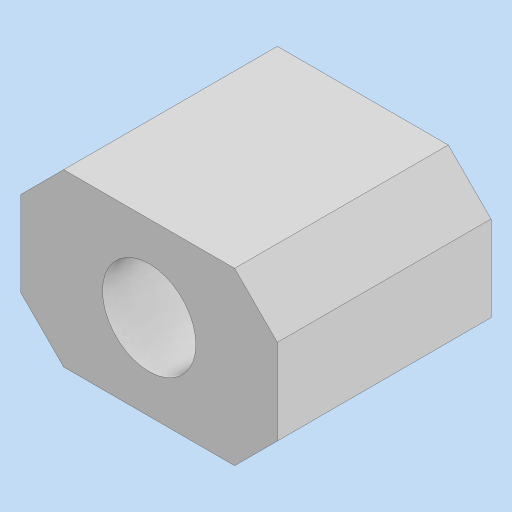
# Autodesk Inventor part: conexion-engrane-hombro
Saved by Autodesk Inventor 2024 (Build 280153000, 153)
## iProperties
Created: 2024-09-11
Part Number: conexion-engrane-hombro
Material: Generic
Document SubType Name: Modeling
Designer: MxMon
Density: 1 g/cm^3
Appearance: Default
Author: MxMon
Autodesk Inventor part; units mm, degrees
ref_plane "YZ Plane" through (0, 0, 0) normal (1, 0, 0) x (0, 1, 0)
ref_plane "XZ Plane" through (0, 0, 0) normal (0, 1, 0) x (-1, 0, 0)
ref_plane "XY Plane" through (0, 0, 0) normal (0, 0, 1) x (1, 0, 0)
sketch "Sketch1" plane through (0, 0, 0) normal (0, 0, 1) x (1, 0, 0)
  line L0 (-6, 4) -> (6, 4)
  line L1 (6, 4) -> (6, -4)
  line L2 (6, -4) -> (-6, -4)
  line L3 (-6, -4) -> (-6, 4)
  line L4 (-6, 4) -> (6, -4) construction
  line L5 (6, 4) -> (-6, -4) construction
  point P0 (0, 0)
  dimension "d0" = 12
  dimension "d1" = 8
  constraints: 12 end point, 2 midpoint, 2 parallel, 1 horizontal, 1 perpendicular
  measures "d0" distance of L1.end L2.end
  measures "d1" distance of L0.end L1.end
extrude "Extrusion1" add sketch "Sketch1" along normal mid plane 10
chamfer "Chamfer1" distance 2 angle 45 4 edges at (6, 4, 0) (-6, 4, 0) (-6, -4, 0) (6, -4, 0)
sketch "Sketch2" plane through (0, 0, -5) normal (0, 0, -1) x (-1, 0, 0)
  circle A0 centre (0, 0) radius 2.1875
  dimension "d7" = 4.375
  constraints: 1 centre point, 1 coincident
  measures "d7" diameter of A0
extrude "Extrusion2" cut sketch "Sketch2" against normal through all
body "Solid1"
